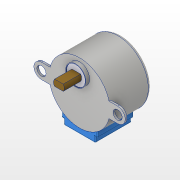
# Autodesk Inventor part: Mini Stepper 5v
Saved by Autodesk Inventor 2022 (Build 260153000, 153)
## iProperties
Created: 2022-09-30
Part Number: Mini Stepper 5v
Material: Generic
Document SubType Name: Modeling
Designer: jeffz
Density: 1 g/cm^3
Appearance: Default
Author: jeffz
Autodesk Inventor part; units mm, degrees
ref_plane "YZ Plane" through (0, 0, 0) normal (1, 0, 0) x (0, 1, 0)
ref_plane "XZ Plane" through (0, 0, 0) normal (0, 1, 0) x (-1, 0, 0)
ref_plane "XY Plane" through (0, 0, 0) normal (0, 0, 1) x (1, 0, 0)
sketch "Sketch1" plane through (0, 0, 0) normal (0, 0, 1) x (1, 0, 0)
  circle A0 centre (0, 0) radius 13.975
  dimension "d0" = 27.95
  constraints: 1 centre point, 1 coincident
  measures "d0" diameter of A0
extrude "Extrusion1" add sketch "Sketch1" along normal blind 19.1
sketch "Sketch2" plane through (0, 0, 19.1) normal (0, 0, 1) x (1, 0, 0)
  circle A0 centre (0, 0) radius 13.975 projected
  line L0 (0, 13.975) -> (0, 3.175)
  circle A1 centre (0, 7.8) radius 4.625
  circle A2 centre (0, 7.8) radius 4.3794
  point P0 (-33.1765, 10.4926)
  dimension "d3" = 10.8
  dimension "d4" = 9.25
  constraints: 2 centre point, 2 end point, 1 vertical, 1 vertical alignment, 1 other
  measures "d3" distance of L0.start L0.end
  measures "d4" diameter of A1
extrude "Extrusion2" add sketch "Sketch2" along normal blind 1.75 contours A1 L0 A2 | L0 A2 A1
sketch "Sketch3" plane through (0, 7.8, 19.1) normal (0, 0, 1) x (1, 0, 0)
  circle A0 centre (0, 0) radius 4.3794 projected
  point P0 (0, -7.8)
extrude "Extrusion3" add sketch "Sketch3" along normal blind 1.5
sketch "Sketch4" plane through (0, 0, 19.1) normal (0, 0, 1) x (1, 0, 0)
  circle A0 centre (0, 7.8) radius 4.3794 projected
  circle A1 centre (0, 0) radius 13.975 projected
  circle A2 centre (0, 7.8) radius 4.625 projected
  line L0 (0, 13.975) -> (0, -0.275)
  circle A3 centre (17.5, 0) radius 2.1
  arc A4 (17.5, -3.475) -> (17.5, 3.475) centre (17.5, 0) ccw
  line L1 (17.5, 3.475) -> (13.5361, 3.475)
  line L2 (17.5, -3.475) -> (13.5361, -3.475)
  circle A5 centre (0, 0) radius 13.975
  circle A6 centre (-17.5, 0) radius 2.1
  arc A7 (-17.5, 3.475) -> (-17.5, -3.475) centre (-17.5, 0) ccw
  line L3 (-17.5, 3.475) -> (-13.5361, 3.475)
  line L4 (-17.5, -3.475) -> (-13.5361, -3.475)
  dimension "d9" = 14.25
  constraints: 10 end point, 9 point on circle, 6 symmetric about line, 4 centre point, 3 coincident, 2 tangent, 1 horizontal, 1 parallel, 1 vertical, 5 other
  measures "d9" distance of L0.start L0.end
extrude "Extrusion4" add sketch "Sketch4" against normal blind 0.85 contours L1 A4 L2 A1 | A1 L4 A7 L3
sketch "Sketch5" plane through (0, 7.8, 20.6) normal (0, 0, 1) x (1, 0, 0)
  circle A0 centre (0, 0) radius 4.3794 projected
  line L0 (-2.0058, -1.45) -> (2.0058, -1.45)
  line L1 (2.0058, 1.45) -> (-2.0058, 1.45)
  arc A1 (-2.0058, 1.45) -> (-2.0058, -1.45) centre (0, 0) ccw
  arc A2 (2.0058, -1.45) -> (2.0058, 1.45) centre (0, 0) ccw
  point P0 (0, -7.8)
  constraints: 4 end point, 4 point on circle, 2 centre point, 1 coincident, 1 parallel
extrude "Extrusion5" add sketch "Sketch5" along normal blind 8 contours A1 L1 A2 L0
sketch "Sketch6" plane through (0, 0, 19.1) normal (0, 0, 1) x (1, 0, 0)
  circle A0 centre (17.5, 0) radius 2.1 projected
  circle A1 centre (-17.5, 0) radius 2.1 projected
  arc A2 (13.5361, 3.475) -> (-13.5361, 3.475) centre (0, 0) ccw projected
  line L0 (-13.5361, 3.475) -> (-17.5, 3.475) projected
  arc A3 (-17.5, 3.475) -> (-17.5, -3.475) centre (-17.5, 0) ccw projected
  line L1 (-17.5, -3.475) -> (-13.5361, -3.475) projected
  arc A4 (-13.5361, -3.475) -> (13.5361, -3.475) centre (0, 0) ccw projected
  line L2 (13.5361, -3.475) -> (17.5, -3.475) projected
  arc A5 (17.5, -3.475) -> (17.5, 3.475) centre (17.5, 0) ccw projected
  line L3 (17.5, 3.475) -> (13.5361, 3.475) projected
  circle A6 centre (0, 7.8) radius 4.625 projected
  line L4 (0, -13.975) -> (0, -16.475)
  line L5 (0, -16.475) -> (-7.25, -16.475)
  line L6 (-7.25, -16.475) -> (-7.25, -13.975)
  line L7 (0, -16.475) -> (7.25, -16.475)
  line L8 (7.25, -16.475) -> (7.25, -13.975)
  line L9 (7.25, -13.975) -> (8.25, -13.975)
  line L10 (8.25, -13.975) -> (8.25, -11.28)
  line L11 (-7.25, -13.975) -> (-8.25, -13.975)
  line L12 (-8.25, -13.975) -> (-8.25, -11.28)
  dimension "d20" = 2.5
  dimension "d21" = 7.25
  dimension "d22" = 7.25
  dimension "d23" = 1
  dimension "d24" = 1
  constraints: 18 end point, 6 perpendicular, 3 point on circle, 1 horizontal, 1 point on line, 1 vertical
  measures "d20" distance of L4.start L4.end
  measures "d21" distance of L4.end L5.end
  measures "d22" distance of L4.end L7.end
  measures "d23" distance of L8.end L9.end
  measures "d24" distance of L6.end L11.end
extrude "Extrusion6" add sketch "Sketch6" against normal blind 16.6 separate body contours L10 L9 L8 L7 L4 A4 | A4 L4 L5 L6 L11 L12
fillet "Fillet1" radius 1.5 1 edges at (-13.975, 0, 0)
sketch "Sketch7" plane through (-7.25, -16.475, 19.1) normal (0, -1, 0) x (1, 0, 0)
  line L0 (0, 0) -> (14.5, 0) projected
  line L1 (7.25, 0) -> (7.25, -2)
  line L2 (7.25, -2) -> (4, -2)
  line L3 (3.25, -2.75) -> (3.25, -2.75)
  line L4 (4, -3.5) -> (10.5, -3.5)
  line L5 (11.25, -2.75) -> (11.25, -2.75)
  line L6 (10.5, -2) -> (7.25, -2)
  arc A0 (10.5, -3.5) -> (11.25, -2.75) centre (10.5, -2.75) ccw
  arc A1 (11.25, -2.75) -> (10.5, -2) centre (10.5, -2.75) ccw
  arc A2 (4, -2) -> (3.25, -2.75) centre (4, -2.75) ccw
  arc A3 (3.25, -2.75) -> (4, -3.5) centre (4, -2.75) ccw
  point P0 (7.25, -19.1)
  point P1 (3.25, -2)
  point P2 (3.25, -3.5)
  point P3 (11.25, -3.5)
  point P4 (11.25, -2)
  dimension "d28" = 2
  dimension "d29" = 4
  dimension "d30" = 1.5
  dimension "d31" = 8
  dimension "d32" = 0.75
  constraints: 12 end point, 9 point on line, 8 point on circle, 8 tangent, 5 perpendicular, 4 centre point, 3 equal radius, 1 midpoint, 1 vertical
  measures "d28" distance of L1.start L1.end
  measures "d29" distance of L1.end point (3.25, -2)
  measures "d30" distance of point (3.25, -2) point (3.25, -3.5)
  measures "d31" distance of point (3.25, -3.5) point (11.25, -3.5)
  measures "d32" radius of A0
extrude "Extrusion7" cut sketch "Sketch7" against normal blind 2 bodies 2
fillet "Fillet2" radius 0.5 4 edges at (8.25, -13.975, 10.8) (7.25, -16.475, 10.8) (-8.25, -13.975, 10.8) (-7.25, -16.475, 10.8)
fillet "Fillet3" radius 0.5 22 edges at (7.25, -14.975, 2.5) (0, -16.475, 2.5) (-7.1036, -16.3286, 2.5) (-7.25, -14.975, 2.5) (7.1036, -16.3286, 2.5) (8.25, -12.3775, 2.5) (7.5, -13.975, 2.5) (8.1036, -13.8286, 2.5) (-8.1036, -13.8286, 2.5) (-8.25, -12.3775, 2.5) (-7.5, -13.975, 2.5) (7.1036, -16.3286, 19.1) (0, -16.475, 19.1) (-7.1036, -16.3286, 19.1) (-7.25, -14.975, 19.1) (7.25, -14.975, 19.1) (7.5, -13.975, 19.1) (8.25, -12.3775, 19.1) (8.1036, -13.8286, 19.1) (-8.25, -12.3775, 19.1) (-7.5, -13.975, 19.1) (-8.1036, -13.8286, 19.1)
body "Solid1"
body "Solid2"
